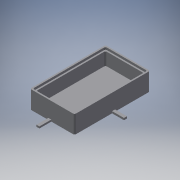
# Autodesk Inventor part: iceTubeClockBase
Saved by Autodesk Inventor 2016 (Build 200138000, 138)
## iProperties
Created: 2016-04-01
Part Number: iceTubeClockBase
Material: Generic
Document SubType Name: Modeling
Designer: boztalay
Density: 1 g/cm^3
Appearance: Default
Author: boztalay
Autodesk Inventor part; units mm, degrees
ref_plane "YZ Plane" through (0, 0, 0) normal (1, 0, 0) x (0, 1, 0)
ref_plane "XZ Plane" through (0, 0, 0) normal (0, 1, 0) x (-1, 0, 0)
ref_plane "XY Plane" through (0, 0, 0) normal (0, 0, 1) x (1, 0, 0)
sketch "Sketch2" plane through (0, 0, 0) normal (0, 1, 0) x (-1, 0, 0)
  line L0 (-47.625, 80.645) -> (47.625, 80.645)
  line L1 (47.625, 80.645) -> (47.625, -80.645)
  line L2 (47.625, -80.645) -> (-47.625, -80.645)
  line L3 (-47.625, -80.645) -> (-47.625, 80.645)
  line L4 (-47.625, 80.645) -> (47.625, -80.645) construction
  line L5 (47.625, 80.645) -> (-47.625, -80.645) construction
  point P0 (0, 0)
  dimension "d6" = 161.29
  dimension "d7" = 95.25
  constraints: 12 end point, 2 midpoint, 2 parallel, 1 horizontal, 1 perpendicular
  measures "d6" distance of L0.end L1.end
  measures "d7" distance of L1.end L2.end
extrude "Extrusion2" add sketch "Sketch2" along normal blind 6.35
sketch "Sketch3" plane through (0, 6.35, 0) normal (0, 1, 0) x (1, 0, 0)
  line L0 (47.625, 80.645) -> (-47.625, 80.645) projected
  line L1 (47.625, -80.645) -> (-47.625, -80.645)
  line L2 (-47.625, -80.645) -> (-47.625, 80.645)
  line L3 (-47.625, 80.645) -> (47.625, 80.645)
  line L4 (47.625, 80.645) -> (47.625, -80.645)
  line L5 (47.625, -80.645) -> (-47.625, 80.645) construction
  line L6 (-47.625, -80.645) -> (47.625, 80.645) construction
  line L7 (41.275, -74.295) -> (-41.275, -74.295)
  line L8 (-41.275, -74.295) -> (-41.275, 74.295)
  line L9 (-41.275, 74.295) -> (41.275, 74.295)
  line L10 (41.275, 74.295) -> (41.275, -74.295)
  line L11 (41.275, -74.295) -> (-41.275, 74.295) construction
  line L12 (-41.275, -74.295) -> (41.275, 74.295) construction
  point P0 (0, 0)
  dimension "d10" = 148.59
  dimension "d11" = 82.55
  constraints: 24 end point, 4 midpoint, 4 parallel, 2 horizontal, 2 perpendicular
  measures "d10" distance of L7.end L8.end
  measures "d11" distance of L8.end L9.end
extrude "Extrusion3" add sketch "Sketch3" along normal blind 31.75
sketch "Sketch6" plane through (0, 38.1, 0) normal (0, 1, 0) x (1, 0, 0)
  line L0 (44.45, -77.47) -> (-44.45, -77.47)
  line L1 (-44.45, -77.47) -> (-44.45, 77.47)
  line L2 (-44.45, 77.47) -> (44.45, 77.47)
  line L3 (44.45, 77.47) -> (44.45, -77.47)
  line L4 (44.45, -77.47) -> (-44.45, 77.47) construction
  line L5 (-44.45, -77.47) -> (44.45, 77.47) construction
  point P0 (0, 0)
  dimension "d29" = 154.94
  dimension "d30" = 88.9
  constraints: 12 end point, 2 midpoint, 2 parallel, 1 horizontal, 1 perpendicular
  measures "d29" distance of L0.end L1.end
  measures "d30" distance of L1.end L2.end
extrude "Extrusion6" cut sketch "Sketch6" against normal blind 4.7625
sketch "Sketch9" plane through (-47.625, 0, -80.645) normal (-1, 0, 0) x (0, 0, 1)
  line L0 (161.29, 0) -> (0, 0) projected
  line L1 (74.8462, 0) -> (81.1962, 0)
  line L2 (81.1962, 0) -> (81.1962, 4.1295)
  line L3 (81.1962, 4.1295) -> (74.8462, 4.1295)
  line L4 (74.8462, 4.1295) -> (74.8462, 0)
  point P0 (80.645, 0)
  dimension "d57" = 6.35
  constraints: 8 end point, 2 parallel, 1 horizontal, 1 perpendicular, 1 point on line
  measures "d57" distance of L2.end L3.end
extrude "Extrusion9" add sketch "Sketch9" along normal blind 25.4
sketch "Sketch10" plane through (-47.625, 0, 80.645) normal (0, 0, 1) x (1, 0, 0)
  line L0 (95.25, 0) -> (0, 0) projected
  line L1 (39.3541, 0) -> (45.7041, 0)
  line L2 (45.7041, 0) -> (45.7041, 3.778)
  line L3 (45.7041, 3.778) -> (39.3541, 3.778)
  line L4 (39.3541, 3.778) -> (39.3541, 0)
  point P0 (47.625, 0)
  dimension "d56" = 6.35
  constraints: 8 end point, 2 parallel, 1 horizontal, 1 perpendicular, 1 point on line
  measures "d56" distance of L2.end L3.end
extrude "Extrusion10" add sketch "Sketch10" along normal blind 25.4
sketch "Sketch11" plane through (47.625, 0, 80.645) normal (1, 0, 0) x (0, 0, -1)
  line L0 (161.29, 0) -> (0, 0) projected
  line L1 (86.4438, 4.1295) -> (86.4438, 0) projected
  line L2 (80.0938, 0) -> (86.4438, 0)
  line L3 (86.4438, 0) -> (86.4438, 4.1295)
  line L4 (86.4438, 4.1295) -> (80.0938, 4.1295)
  line L5 (80.0938, 4.1295) -> (80.0938, 0)
  point P0 (80.645, 0)
  dimension "d55" = 6.35
  constraints: 8 end point, 2 parallel, 1 horizontal, 1 perpendicular, 1 point on line
  measures "d55" distance of L1.start L4.end
extrude "Extrusion11" add sketch "Sketch11" along normal blind 25.4
sketch "Sketch12" plane through (47.625, 0, -80.645) normal (0, 0, -1) x (-1, 0, 0)
  line L0 (41.275, 0) -> (47.625, 0)
  line L1 (47.625, 0) -> (47.625, 3.778)
  line L2 (47.625, 3.778) -> (41.275, 3.778)
  line L3 (41.275, 3.778) -> (41.275, 0)
  dimension "d54" = 6.35
  constraints: 8 end point, 2 parallel, 1 coincident, 1 horizontal, 1 perpendicular
  measures "d54" distance of L1.end L2.end
extrude "Extrusion12" add sketch "Sketch12" along normal blind 25.4
fillet "Fillet1" radius 3.175 12 edges at (47.625, 19.05, 80.645) (47.625, 19.05, -80.645) (-47.625, 19.05, -80.645) (-47.625, 19.05, 80.645) (44.45, 35.7187, -77.47) (41.275, 19.8437, -74.295) (-41.275, 19.8437, -74.295) (-44.45, 35.7187, -77.47) (-41.275, 19.8437, 74.295) (-44.45, 35.7187, 77.47) (41.275, 19.8437, 74.295) (44.45, 35.7187, 77.47)
sketch "Sketch13" plane through (0, 0, 0) normal (0, -1, 0) x (1, 0, 0)
  line L0 (-24.765, 53.975) -> (24.765, 53.975) construction
  line L1 (24.765, 53.975) -> (24.765, -53.975) construction
  line L2 (24.765, -53.975) -> (-24.765, -53.975) construction
  line L3 (-24.765, -53.975) -> (-24.765, 53.975) construction
  line L4 (-24.765, 53.975) -> (24.765, -53.975) construction
  line L5 (24.765, 53.975) -> (-24.765, -53.975) construction
  circle A0 centre (24.765, 53.975) radius 10.9982
  circle A1 centre (24.765, 22.225) radius 10.9982
  circle A2 centre (24.765, -22.225) radius 10.9982
  circle A3 centre (24.765, -53.975) radius 10.9982
  line L6 (-47.625, -5.7988) -> (-47.625, -77.47) construction
  point P0 (0, 0)
  dimension "d58" = 21.9964
  dimension "d59" = 21.9964
  dimension "d60" = 21.9964
  dimension "d61" = 21.9964
  dimension "d62" = 31.75
  dimension "d63" = 44.45
  dimension "d64" = 31.75
  dimension "d66" = 72.39
  constraints: 12 end point, 4 centre point, 2 coincident, 2 midpoint, 2 parallel, 2 point on line, 1 horizontal, 1 perpendicular
  measures "d58" diameter of A0
  measures "d59" diameter of A1
  measures "d60" diameter of A2
  measures "d61" diameter of A3
  measures "d62" distance of A1.centre L0.end
  measures "d63" distance of A2.centre A1.centre
  measures "d64" distance of L1.end A2.centre
  measures "d66" distance between parallel lines of L6 L1
extrude "Extrusion13" cut sketch "Sketch13" against normal up to next
body "Solid2"
